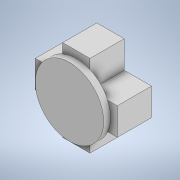
# Autodesk Inventor part: PlusBtn
Saved by Autodesk Inventor 2020.1 (Build 241239000, 239)
## iProperties
Created: 2019-09-04
Part Number: PlusBtn
Material: Generic
Document SubType Name: Modeling
Designer: matteo.spadetto-1
Density: 1 g/cm^3
Appearance: Default
Author: matteo.spadetto-1
Autodesk Inventor part; units mm, degrees
ref_plane "YZ Plane" through (0, 0, 0) normal (1, 0, 0) x (0, 1, 0)
ref_plane "XZ Plane" through (0, 0, 0) normal (0, 1, 0) x (-1, 0, 0)
ref_plane "XY Plane" through (0, 0, 0) normal (0, 0, 1) x (1, 0, 0)
sketch "Sketch1" plane through (0, 0, 0) normal (0, 0, 1) x (1, 0, 0)
  line L0 (6, 12) -> (4, 12)
  line L1 (6, 12) -> (8, 12)
  line L2 (12, 6) -> (12, 8)
  line L3 (12, 6) -> (12, 4)
  line L4 (0, 6) -> (0, 8)
  line L5 (0, 6) -> (0, 4)
  line L6 (6, 0) -> (8, 0)
  line L7 (6, 0) -> (4, 0)
  line L8 (4, 0) -> (4, 4)
  line L9 (4, 4) -> (0, 4)
  line L10 (0, 8) -> (4, 8)
  line L11 (4, 8) -> (4, 12)
  line L12 (8, 12) -> (8, 8)
  line L13 (8, 8) -> (12, 8)
  line L14 (8, 0) -> (8, 4)
  line L15 (8, 4) -> (12, 4)
  point P0 (0, 0)
  dimension "d2" = 2
  dimension "d3" = 2
  dimension "d4" = 2
  dimension "d5" = 2
  dimension "d6" = 2
  dimension "d7" = 2
  dimension "d8" = 2
  dimension "d9" = 2
  constraints: 32 end point, 5 perpendicular, 1 horizontal, 1 point on line, 1 vertical
  measures "d2" distance of L0.start L0.end
  measures "d3" distance of L0.start L1.end
  measures "d4" distance of L2.start L2.end
  measures "d5" distance of L2.start L3.end
  measures "d6" distance of L4.start L4.end
  measures "d7" distance of L4.start L5.end
  measures "d8" distance of L6.start L6.end
  measures "d9" distance of L6.start L7.end
extrude "Extrusion1" add sketch "Sketch1" along normal blind 5
sketch "Sketch2" plane through (0, 0, 5) normal (0, 0, 1) x (1, 0, 0)
  line L0 (0, 8) -> (0, 4) projected
  line L1 (0, 6) -> (12, 6)
  line L2 (12, 4) -> (12, 8) projected
  line L3 (8, 12) -> (4, 12) projected
  line L4 (6, 12) -> (6, 0)
  circle A0 centre (6, 6) radius 5
  point P0 (0, 0)
  dimension "d12" = 10
  constraints: 4 end point, 4 midpoint, 1 centre point, 1 vertical
  measures "d12" diameter of A0
extrude "Extrusion2" add sketch "Sketch2" along normal blind 1
body "Solid1"
